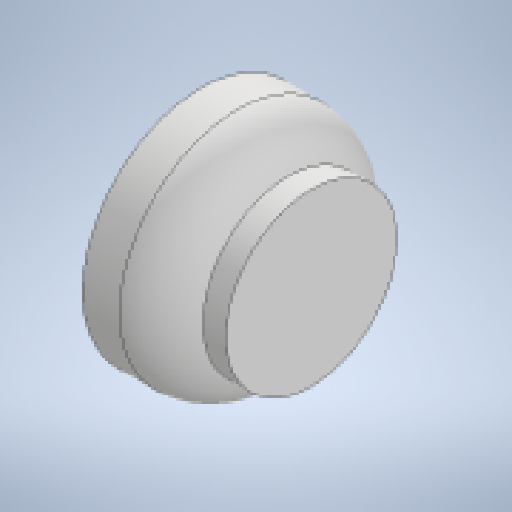
# Autodesk Inventor part: TheLens
Saved by Autodesk Inventor 2025.1 (Build 291241000, 241)
## iProperties
Created: 2025-06-16
Part Number: TheLens
Material: Generic
Document SubType Name: Modeling
Designer: User
Density: 1 g/cm^3
Appearance: Default
Author: User
Autodesk Inventor part; units mm, degrees
ref_plane "YZ Plane" through (0, 0, 0) normal (1, 0, 0) x (0, 1, 0)
ref_plane "XZ Plane" through (0, 0, 0) normal (0, 1, 0) x (-1, 0, 0)
ref_plane "XY Plane" through (0, 0, 0) normal (0, 0, 1) x (1, 0, 0)
sketch "Sketch1" plane through (0, 0, 0) normal (0, 0, 1) x (1, 0, 0)
  arc A0 (-73.0041, 39.7342) -> (-88.7899, 41.7717) centre (-81.1499, 38.7933) ccw projected
  line L0 (-92.3771, 6.5) -> (-92.3771, -6.5) projected
  line L1 (-92.3771, 0) -> (-118.3771, 0)
  line L2 (-97.8771, -18.5) -> (-97.8771, 18.5) projected
  line L3 (-97.8771, 0) -> (-121.8771, 0)
  line L4 (-121.8771, 0) -> (-121.8771, -25.5)
  line L5 (-97.8771, 0) -> (-97.8771, -18.5)
  line L6 (-97.8771, -18.5) -> (-102.8771, -18.5)
  line L7 (-121.8771, -25.5) -> (-113.8771, -25.5)
  arc A1 (-113.8771, -25.5) -> (-102.8771, -18.5) centre (-113.8771, -13.3571) ccw
  line L8 (-97.8771, -18.5) -> (-97.8771, 0)
  point P0 (0, 0)
  point P1 (-97.8771, 0)
  dimension "d1" = 24
  dimension "d2" = 25.5
  dimension "d3" = 5
  dimension "d4" = 8
  constraints: 14 end point, 3 horizontal, 2 collinear, 2 midpoint, 2 point on circle, 1 centre point, 1 point on line, 1 tangent, 1 vertical
  measures "d1" distance of L3.start L3.end
  measures "d2" distance of L3.end L4.end
  measures "d3" distance of L2.start L6.end
  measures "d4" distance of L4.end L7.end
revolve "Revolution1" add sketch "Sketch1" angle 360 about axis through (-92.3771, 0, 0) along (-1, 0, 0)
body "Solid1"
